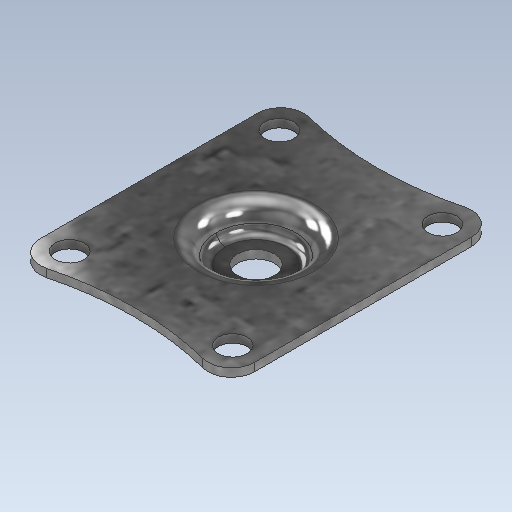
# Autodesk Inventor part: Wheel 75 mm - Part 6
Saved by Autodesk Inventor 2020 (Build 240168000, 168)
## iProperties
Created: 2022-11-13
Part Number: Wheel 75 mm - Part 6
Material: Generic
Document SubType Name: Modeling
Designer: saad.nashed
Density: 1 g/cm^3
Appearance: Steel Galvanized
d15: 8.000 mm
d4: 45.000 mm
d5: 35.000 mm
Author: saad.nashed
Autodesk Inventor part; units mm, degrees
ref_plane "YZ Plane" through (0, 0, 0) normal (1, 0, 0) x (0, 1, 0)
ref_plane "XZ Plane" through (0, 0, 0) normal (0, 1, 0) x (-1, 0, 0)
ref_plane "XY Plane" through (0, 0, 0) normal (0, 0, 1) x (1, 0, 0)
sketch "Sketch1" plane through (0, 0, 0) normal (0, 1, 0) x (-1, 0, 0)
  line L0 (-23, 23.29) -> (-23, -23.29)
  line L1 (23, -23.29) -> (23, 23.29)
  line L2 (0, 0) -> (0, -50.5577)
  line L3 (0, 0) -> (-7.5284, 0)
  arc A0 (16.748, -28.1307) -> (-16.748, -28.1307) centre (0, -92.8874) ccw
  arc A1 (-16.748, 28.1307) -> (16.748, 28.1307) centre (0, 92.8874) ccw
  arc A2 (-16.748, 28.1307) -> (-23, 23.29) centre (-18, 23.29) ccw
  arc A3 (-23, -23.29) -> (-16.748, -28.1307) centre (-18, -23.29) ccw
  arc A4 (16.748, -28.1307) -> (23, -23.29) centre (18, -23.29) ccw
  arc A5 (23, 23.29) -> (16.748, 28.1307) centre (18, 23.29) ccw
  line L4 (61.758, -28.29) -> (80.0321, -28.29)
  line L5 (64.4221, 28.29) -> (84.7267, 28.29)
  circle A6 centre (-17.5, -22.5) radius 3.1
  circle A7 centre (17.5, 22.5) radius 3.1
  circle A8 centre (17.5, -22.5) radius 3.1
  circle A9 centre (-17.5, 22.5) radius 3.1
  circle A10 centre (0, 0) radius 8.5
  circle A11 centre (0, 0) radius 4
  dimension "d0" = 52
  dimension "d1" = 46
  dimension "d2" = 5
  dimension "d3" = 56.58
  dimension "d4" = 45
  dimension "d5" = 35
  dimension "d6" = 6.2
  dimension "d9" = 17
  dimension "d15" = 8
  constraints: 12 centre point, 12 end point, 12 point on circle, 10 tangent, 3 equal radius, 3 horizontal, 2 coincident, 1 parallel, 1 point on line, 1 vertical, 5 other
  measures "d1" distance between parallel lines of L0 L1
  measures "d2" radius of A2
  measures "d3" distance between parallel lines of L5 L4
  measures "d4" distance of A7.centre A8.centre
  measures "d5" distance of A6.centre A8.centre
  measures "d6" diameter of A6
  measures "d9" diameter of A10
  measures "d15" diameter of A11
extrude "Extrusion1" add sketch "Sketch1" against normal blind 10 contours A2 A1 A5 L1 A4 A0 A3 L0 | L3 A11 L2 | L2 A11 L3 | A6 | A7 | A8 | A9 | A10
extrude "Extrusion2" cut sketch "Sketch1" against normal blind 5 contours L3 A11 L2 | L2 A11 L3 | A10
fillet "Fillet1" radius 4 1 edges at (8.5, 0, 0)
fillet "Fillet2" radius 2 1 edges at (8.5, -5, 0)
shell "Shell1" thickness 1.75 removed faces 9 at (11.424, -10, -7.7633) at (22.3091, -6.6667, 25.8261) at (17.1192, -6.6667, -28.2118) at (-13.0815, -3.3333, 27.2917) at (-13.0815, -6.6667, -27.2917) at (-22.1041, -6.6667, 26.146) at (-22.3091, -6.6667, -25.8261) at (-23, -3.3333, -7.7633) at (23, -3.3333, 7.7633)
extrude "Extrusion3" cut sketch "Sketch1" against normal through all contours L3 A11 L2 | L2 A11 L3 | A6 | A7 | A8 | A9
equation "\"d15\" = 2 * d25"
equation "\"d25\" = 4"
body "Solid1"
